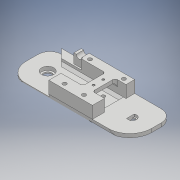
# Autodesk Inventor part: phalanx 1 R F5
Saved by Autodesk Inventor 2017 (Build 210142000, 142)
## iProperties
Created: 2018-07-24
Part Number: phalanx 1 R F5
Material: Generic
Document SubType Name: Modeling
Designer: jakub.tomczynski
Density: 1 g/cm^3
Appearance: Default
Author: jakub.tomczynski
## iProperties of the stored document phalanx 1 R F5_3DPrint.ipt
Created: 2018-09-03
Part Number: phalanx 1 R F5_3DPrint
Material: Generic
Document SubType Name: Modeling
Designer: jakub.tomczynski
Density: 1 g/cm^3
Appearance: Default
Author: jakub.tomczynski
Autodesk Inventor part; units mm, degrees
ref_plane "YZ Plane" through (0, 0, 0) normal (1, 0, 0) x (0, 1, 0)
ref_plane "XZ Plane" through (0, 0, 0) normal (0, 1, 0) x (-1, 0, 0)
ref_plane "XY Plane" through (0, 0, 0) normal (0, 0, 1) x (1, 0, 0)
sketch "axes" plane through (0, 0, 0) normal (0, 0, 1) x (1, 0, 0)
  point P0 (0, 0)
  point P1 (-35, 0)
  point P2 (0, 0)
  dimension "d0" = 35
  constraints: 1 coincident, 1 horizontal alignment
  measures "d0" distance of point (0, 0) point (-35, 0)
sketch "tendon anchors" plane through (0, 0, 0) normal (0, 0, 1) x (1, 0, 0)
  line L0 (-8.2564, 0) -> (0, 0) construction
  line L1 (0, 0) -> (-7.5, -7.5) construction
  line L2 (-27.0254, 0) -> (-35, 0) construction
  line L3 (-35, 0) -> (-25.5, -5.5) construction
  dimension "d136" = 7.5
  dimension "d137" = 7.5
  dimension "d138" = 5.5
  dimension "d139" = 9.5
  constraints: 8 end point, 2 coincident, 2 horizontal
  measures "d136" distance from line of L1.end L0
  measures "d137" horizontal distance of L1.end point (0, 0)
  measures "d138" vertical distance of L3.end point (-35, 0)
  measures "d139" horizontal distance of L3.end point (-35, 0)
sketch "Sketch3" plane through (0, 0, 0) normal (0, 0, 1) x (1, 0, 0)
  line L0 (-43, 9) -> (8, 9)
  line L1 (8, 9) -> (8, -9)
  line L2 (8, -9) -> (-43, -9)
  line L3 (-43, -9) -> (-43, 9)
  point P0 (0, 0)
  point P1 (8, 0)
  point P2 (-35, 0)
  dimension "d1" = 18
  dimension "d2" = 8
  dimension "d3" = 8
  constraints: 8 end point, 2 parallel, 1 horizontal, 1 horizontal alignment, 1 midpoint, 1 perpendicular
  measures "d1" distance between parallel lines of L2 L0
  measures "d2" distance from line of L1 point (0, 0)
  measures "d3" distance from line of point (-35, 0) L3
extrude "base plate" add sketch "Sketch3" along normal blind 2
sketch "Sketch4" plane through (0, 0, 2) normal (0, 0, 1) x (1, 0, 0)
  line L0 (8, 9) -> (-43, 9) projected
  line L1 (-43, 9) -> (-43, -9) projected
  line L2 (-43, -9) -> (8, -9) projected
  line L3 (8, -9) -> (8, 9) projected
  line L4 (-26.5, 9) -> (-8, 9)
  line L5 (-8, 9) -> (-8, 5.4)
  line L6 (-8, 5.4) -> (-26.5, 5.4)
  line L7 (-26.5, 5.4) -> (-26.5, 9)
  line L8 (-25.5, -9) -> (-7.5, -9)
  line L9 (-7.5, -9) -> (-7.5, -4)
  line L10 (-7.5, -4) -> (-25.5, -4)
  line L11 (-25.5, -4) -> (-25.5, -9)
  point P0 (0, 0)
  point P1 (-25.5, -5.5)
  point P2 (-7.5, -7.5)
  dimension "d6" = 5
  dimension "d7" = 3.6
  dimension "d8" = 16.5
  dimension "d9" = 16
  constraints: 16 end point, 4 parallel, 2 horizontal, 2 perpendicular, 2 point on line, 2 vertical alignment
  measures "d6" distance between parallel lines of L2 L10
  measures "d7" distance between parallel lines of L6 L0
  measures "d8" distance between parallel lines of L7 L1
  measures "d9" distance between parallel lines of L3 L5
extrude "walls" add sketch "Sketch4" along normal blind 4.5 contours L5 L6 L7 L0 | L2 L11 L10 L9
sketch "Sketch5" plane through (0, 0, 2) normal (0, 0, 1) x (1, 0, 0)
  point P0 (0, 0)
  point P1 (-35, 0)
  point P2 (0, 0)
hole "joint bearings" at (-35, 0, 2) direction (0, 0, -1) diameter 3.5 end through all counterbore diameter 5 counterbore depth 1.5
fillet "front top" radius 5 1 edges at (-43, 9, 1)
fillet "front bottom" radius 8 1 edges at (-43, -9, 1)
sketch "Sketch7" plane through (0, 0, 2) normal (0, 0, 1) x (1, 0, 0)
  circle A0 centre (-35, 0) radius 4
  line L0 (-26.5, 9) -> (-38, 9) projected
  arc A1 (-38, 9) -> (-43, 4) centre (-38, 4) ccw projected
  line L1 (-26.5, 5.4) -> (-26.5, 9) projected
  line L2 (-38.3321, 8.989) -> (-32.1716, 2.8284)
  line L3 (-35, 0) -> (-47.831, 0) construction
  line L4 (-26.5, 5.4) -> (-34.7431, 5.4)
  point P0 (0, 0)
  dimension "d33" = 8
  dimension "d34" = 45
  constraints: 6 end point, 2 horizontal, 1 coincident, 1 point on circle, 1 point on line, 4 other
  measures "d34" angle of L3 L2
extrude "extension endstop" add sketch "Sketch7" along normal blind 2 contours L2 A1 L0 L1 L4
sketch "Sketch8" plane through (0, 0, 2) normal (0, 0, 1) x (1, 0, 0)
  point P0 (0, 0)
  point P1 (-35, 0)
  point P2 (-14.5, 2.5)
  point P3 (-14.5, 2.5)
  point P4 (-14.5, -1.5)
  dimension "d41" = 20.5
  dimension "d73" = 2.5
  dimension "d127" = 1.5
  constraints: 1 coincident, 1 vertical alignment
  measures "d41" horizontal distance of point (-14.5, 2.5) point (-35, 0)
  measures "d73" vertical distance of point (-14.5, 2.5) point (-35, 0)
  measures "d127" vertical distance of point (-14.5, -1.5) point (-35, 0)
hole "spring pin" at (-14.5, 2.5, 2) at (-14.5, -1.5, 2) direction (0, 0, -1) diameter 1.5 end through all
sketch "Sketch10" plane through (0, 0, 2) normal (0, 0, 1) x (1, 0, 0)
  line L0 (-9, -9) -> (8, -9)
  line L1 (8, -9) -> (8, 9)
  line L2 (8, 9) -> (-9, 9)
  line L3 (-9, 9) -> (-9, -9)
  point P0 (0, 0)
  point P1 (-8, 9)
  dimension "d126" = 17
  constraints: 8 end point, 2 parallel, 1 horizontal, 1 perpendicular
  measures "d126" distance between parallel lines of L3 L1
extrude "Extrusion4" add sketch "Sketch10" along normal blind 1
sketch "Sketch11" plane through (0, 0, 0) normal (0, 0, -1) x (-1, 0, 0)
  circle A0 centre (0, 0) radius 9
  line L0 (0, 9) -> (-9, 9)
  line L1 (-9, 9) -> (-9, -9)
  line L2 (-9, -9) -> (9, -9)
  line L3 (9, -9) -> (9, 0)
  dimension "d57" = 18
  constraints: 8 end point, 4 tangent, 3 perpendicular, 2 point on circle, 1 centre point, 1 coincident, 1 horizontal
  measures "d57" diameter of A0
extrude "Extrusion5" cut sketch "Sketch11" against normal blind 1.5
fillet "Fillet5" radius 1 2 edges at (0, 9, 0.75) (-9, -9, 0.75)
fillet "Fillet6" radius 5 1 edges at (8, 9, 2.25)
fillet "Fillet7" radius 9 1 edges at (8, -9, 2.25)
sketch "Sketch12" plane through (0, 0, 3) normal (0, 0, 1) x (1, 0, 0)
  circle A0 centre (0, 0) radius 1.75
  line L0 (-0.75, -1.5811) -> (-0.75, 1.5811)
  dimension "d63" = 3.5
  dimension "d140" = 0.75
  constraints: 2 end point, 2 point on circle, 1 centre point, 1 coincident, 1 vertical
  measures "d63" diameter of A0
  measures "d140" distance from line of point (0, 0) L0
extrude "Extrusion6" cut sketch "Sketch12" against normal blind 1 contours A0 L0 picked at (0.0833, 0)
sketch "Sketch18" plane through (0, 0, 6.5) normal (0, 0, 1) x (1, 0, 0)
  line L0 (-26.5, 9) -> (-26.5, 5.4) projected
  line L1 (-26.5, 5.4) -> (-8, 5.4) projected
  line L2 (-8, 5.4) -> (-8, 9) projected
  line L3 (-8, 9) -> (-26.5, 9) projected
  line L4 (-25.5, -9) -> (-7.5, -9) projected
  line L5 (-7.5, -9) -> (-7.5, -4) projected
  line L6 (-7.5, -4) -> (-25.5, -4) projected
  line L7 (-25.5, -4) -> (-25.5, -9) projected
  circle A0 centre (-14.5, 2.5) radius 0.75 projected
  line L8 (-16.5, 5.4) -> (-12.5, 5.4)
  line L9 (-12.5, 5.4) -> (-12.5, -4)
  line L10 (-12.5, -4) -> (-16.5, -4)
  line L11 (-16.5, -4) -> (-16.5, 5.4)
  line L12 (-14.5, 2.5) -> (-14.5, -2.026) construction
  point P0 (0, 0)
  dimension "d105" = 4
  constraints: 10 end point, 2 parallel, 2 point on line, 1 horizontal, 1 perpendicular, 1 vertical, 1 other
  measures "d105" distance between parallel lines of L9 L11
extrude "Extrusion8" add sketch "Sketch18" along normal blind 1.5 contours L3 L2 L1 L0 | L1 L9 L6 L11 | L6 L5 L4 L7 | A0
sketch "Sketch19" plane through (0, 0, 6.5) normal (0, 0, -1) x (-1, 0, 0)
  circle A0 centre (14.5, 2.5) radius 0.75 projected
  circle A1 centre (14.5, -1.5) radius 0.75 projected
  point P0 (0, 0)
hole "spring pins support" at (-14.5, 2.5, 6.5) at (-14.5, -1.5, 6.5) direction (0, 0, 1) diameter 1 end through all counterbore diameter 1.5 counterbore depth 1.25
sketch "Sketch14" plane through (0, 0, 3) normal (0, 0, 1) x (1, 0, 0)
  line L0 (-0.75, -1.5811) -> (-0.75, 1.5811) projected
  arc A0 (-0.75, -1) -> (-0.75, 1) centre (0, 0) ccw
  dimension "d133" = 2.5
  constraints: 2 point on circle, 2 point on line, 1 centre point, 1 coincident
  measures "d133" diameter of A0
extrude "Extrusion11" cut sketch "Sketch14" against normal through all
sketch "Sketch17" plane through (0, 0, 8) normal (0, 0, 1) x (1, 0, 0)
  point P0 (5, 0)
  point P1 (-21, -7)
  point P2 (-13, -7)
  point P3 (-24.5, 7)
  point P4 (-10.5, 7)
  point P5 (-35, 0)
  point P6 (0, 0)
  point P7 (-35, 0)
  point P8 (0, 0)
  dimension "d92" = 7
  dimension "d93" = 7
  dimension "d94" = 10.5
  dimension "d95" = 10.5
  dimension "d96" = 14
  dimension "d97" = 13
  constraints: 2 coincident, 2 horizontal alignment
  measures "d92" vertical distance of point (5, 0) point (-10.5, 7)
  measures "d93" vertical distance of point (0, 0) point (-13, -7)
  measures "d94" horizontal distance of point (-24.5, 7) point (-35, 0)
  measures "d95" horizontal distance of point (0, 0) point (-10.5, 7)
  measures "d96" horizontal distance of point (-21, -7) point (-35, 0)
  measures "d97" horizontal distance of point (0, 0) point (-13, -7)
hole "mounting" at (-24.5, 7, 8) at (-10.5, 7, 8) at (-21, -7, 8) at (-13, -7, 8) direction (0, 0, -1) diameter 1.6 depth 6 tip angle 118
sketch "Sketch20" plane through (-43, 4, 0) normal (-1, 0, 0) x (0, 0, 1)
  line L0 (3, 5) -> (20, 5)
  line L1 (20, 5) -> (20, -13)
  line L2 (20, -13) -> (3, -13)
  line L3 (0, -10) -> (0, 2)
  arc A0 (3, 5) -> (0, 2) centre (3, 2) ccw
  arc A1 (0, -10) -> (3, -13) centre (3, -10) ccw
  point P0 (0, -4)
  point P1 (0, 5)
  point P2 (0, -13)
  point P3 (0, -13)
  dimension "d115" = 20
  dimension "d116" = 3
  constraints: 8 end point, 4 point on circle, 4 point on line, 4 tangent, 2 centre point, 2 parallel, 1 coincident, 1 equal radius, 1 horizontal, 1 perpendicular
  measures "d115" distance between parallel lines of L3 L1
  measures "d116" radius of A0
extrude "side fillet" cut sketch "Sketch20" against normal through all keep common part
fillet "Fillet8" radius 1 5 edges at (-39.0048, -7.9255, 0.6994) (-43, 1.5, 0) (-42.8945, 5.0215, 0) (-41.0629, 7.9521, 0.722) (-42.5485, -3.6495, 0)
sketch "Sketch21" plane through (-38, 9, 4) normal (0, 1, 0) x (1, 0, 0)
  line L0 (11.5, 0) -> (0, 0) projected
  line L1 (11.5, 0) -> (11.5, -4) projected
  line L2 (10, -4) -> (10, -4) construction
  line L3 (11.15, -4) -> (11.15, -4)
  line L4 (8.85, -4) -> (8.85, -4)
  arc A0 (8.85, -4) -> (11.15, -4) centre (10, -4) ccw
  arc A1 (11.15, -4) -> (8.85, -4) centre (10, -4) ccw
  line L5 (8.85, -4) -> (7.85, -4)
  line L6 (7.85, -4) -> (7.85, 0)
  line L7 (11.15, -4) -> (11.5, -4)
  point P0 (38, 4)
  point P1 (10, -3.75)
  point P2 (3, 4)
  dimension "d120" = 2.3
  dimension "d121" = 7
  dimension "d122" = 0
  dimension "d123" = 1
  constraints: 14 end point, 4 point on circle, 4 tangent, 2 centre point, 2 horizontal, 2 perpendicular, 2 point on line, 1 horizontal alignment, 1 parallel
  measures "d120" distance between parallel lines of L4 L3
  measures "d121" distance from line of point (3, 4) L2
  measures "d122" distance of L2.end L2.start
  measures "d123" distance between parallel lines of L6 L4
extrude "cable clip" add sketch "Sketch21" against normal blind 3 contours L1 L7 A1 L5 L6 L0
chamfer "Chamfer1" distance 1 angle 45 3 edges at (-9, 0.7, 2) (-21.8716, 5.4, 2) (-17.25, -4, 2)
fillet "Fillet9" radius 1 4 edges at (-16.5, 5.4, 7.25) (-12.5, 5.4, 7.25) (-12.5, -4, 7.25) (-16.5, -4, 7.25)
fillet "Fillet10" radius 1 4 edges at (-17, -4, 6.5) (-12, -4, 6.5) (-12, 5.4, 6.5) (-17, 5.4, 6.5)
equation "\"d0\" = MCP_PIP_length"
equation "\"d41\" = PIP_spring_length"
equation "\"MCP_PIP_length\" = F5_MCP_PIP_length"
equation "\"PIP_spring_length\" = F5_PIP_spring_length"
equation "\"F5_MCP_PIP_length\" = 35"
equation "\"F5_PIP_spring_length\" = 20.5"
body "Solid1"
